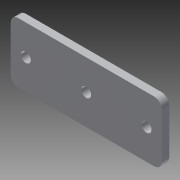
# Autodesk Inventor part: Spacer 4
Saved by Autodesk Inventor 2014 (Build 180170000, 170)
## iProperties
Created: 2014-01-17
Part Number: Spacer 4
Material: Aluminum 6061
Document SubType Name: Modeling
Designer: Michael
Density: 2.71 g/cm^3
Appearance: Aluminum - Flat
Author: Michael
Autodesk Inventor part; units mm, degrees
ref_plane "YZ Plane" through (0, 0, 0) normal (1, 0, 0) x (0, 1, 0)
ref_plane "XZ Plane" through (0, 0, 0) normal (0, 1, 0) x (-1, 0, 0)
ref_plane "XY Plane" through (0, 0, 0) normal (0, 0, 1) x (1, 0, 0)
sketch "Sketch1" plane through (0, 0, 0) normal (0, 0, 1) x (1, 0, 0)
  line L0 (3.175, 0) -> (60.325, 0)
  line L1 (63.5, 3.175) -> (63.5, 22.225)
  line L2 (60.325, 25.4) -> (3.175, 25.4)
  line L3 (0, 22.225) -> (0, 3.175)
  circle A0 centre (6.35, 12.7) radius 2.0701
  line L4 (0, 12.7) -> (63.5, 12.7) construction
  circle A1 centre (31.75, 12.7) radius 2.0701
  circle A2 centre (57.15, 12.7) radius 2.0701
  arc A3 (3.175, 25.4) -> (0, 22.225) centre (3.175, 22.225) ccw
  arc A4 (63.5, 22.225) -> (60.325, 25.4) centre (60.325, 22.225) ccw
  arc A5 (60.325, 0) -> (63.5, 3.175) centre (60.325, 3.175) ccw
  arc A6 (0, 3.175) -> (3.175, 0) centre (3.175, 3.175) ccw
  point P0 (0, 0)
  point P1 (63.5, 25.4)
  point P2 (63.5, 0)
  point P3 (0, 25.4)
  dimension "d0" = 63.5
  dimension "d1" = 25.4
  dimension "d2" = 6.35
  dimension "d3" = 4.1402
  dimension "d6" = 25.4
  dimension "d11" = 3.175
  constraints: 10 end point, 9 point on line, 8 point on circle, 8 tangent, 7 centre point, 3 equal radius, 2 horizontal, 2 midpoint, 2 parallel, 1 perpendicular, 4 other
  measures "d0" distance of point (0, 25.4) point (63.5, 25.4)
  measures "d1" distance of point (63.5, 25.4) point (63.5, 0)
  measures "d2" distance from line of L3 A0.centre
  measures "d3" diameter of A0
  measures "d6" distance of A0.centre A1.centre
  measures "d11" radius of A3
extrude "Extrusion1" add sketch "Sketch1" along normal blind 3.175
body "Solid1"
